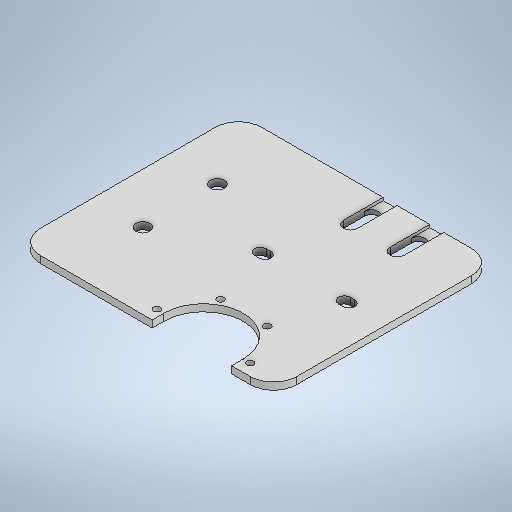
# Autodesk Inventor part: TopMount
Saved by Autodesk Inventor 2025.2 (Build 292293000, 293)
## iProperties
Created: 2025-07-18
Part Number: TopMount
Material: Generic
Document SubType Name: Modeling
Designer: Simon
Density: 1 g/cm^3
Appearance: Default
Author: Simon
Autodesk Inventor part; units mm, degrees
ref_plane "YZ Plane" through (0, 0, 0) normal (1, 0, 0) x (0, 1, 0)
ref_plane "XZ Plane" through (0, 0, 0) normal (0, 1, 0) x (-1, 0, 0)
ref_plane "XY Plane" through (0, 0, 0) normal (0, 0, 1) x (1, 0, 0)
sketch "Sketch1" plane through (0, 0, 0) normal (0, 1, 0) x (-1, 0, 0)
  line L0 (-75, 47.5) -> (75, 47.5)
  line L1 (75, 47.5) -> (75, -47.5)
  line L2 (75, -47.5) -> (-75, -47.5)
  line L3 (-75, -47.5) -> (-75, 47.5)
  line L4 (-75, 47.5) -> (75, -47.5) construction
  line L5 (75, 47.5) -> (-75, -47.5) construction
  point P0 (0, 0)
  dimension "d0" = 150
  dimension "d1" = 95
  constraints: 12 end point, 2 midpoint, 2 parallel, 1 horizontal, 1 perpendicular
  measures "d0" distance of L1.end L2.end
  measures "d1" distance of L0.end L1.end
extrude "Extrusion1" add sketch "Sketch1" along normal blind 3
sketch "Sketch4" plane through (0, 3, 0) normal (0, 1, 0) x (1, 0, 0)
  line L0 (75, 47.5) -> (-75, 47.5) projected
  line L1 (-10, 47.5) -> (10, 47.5)
  line L2 (10, 47.5) -> (10, 27.5)
  line L3 (-10, 47.5) -> (-10, 27.5)
  line L4 (-10, 27.5) -> (10, 27.5)
  line L5 (-13, 47.5) -> (-7, 47.5)
  line L6 (7, 47.5) -> (13, 47.5)
  line L7 (-10, 47.5) -> (-10, 42.5)
  line L8 (10, 47.5) -> (10, 42.5)
  line L9 (-10, 42.5) -> (-10, 39.5)
  line L10 (10, 42.5) -> (10, 39.5)
  line L11 (-10, 27.5) -> (-10, 30.5)
  line L12 (10, 27.5) -> (10, 30.5)
  circle A0 centre (-10, 30.5) radius 3
  circle A1 centre (10, 30.5) radius 3
  circle A2 centre (-10, 39.5) radius 3
  circle A3 centre (10, 39.5) radius 3
  line L13 (-13, 39.5) -> (-13, 30.5)
  line L14 (-7, 39.5) -> (-7, 30.5)
  line L15 (7, 39.5) -> (7, 30.5)
  line L16 (13, 39.5) -> (13, 30.5)
  line L17 (-10, 27.5) -> (-7, 27.5)
  line L18 (-7, 27.5) -> (-7, 47.5)
  line L19 (-7, 47.5) -> (-10, 47.5)
  line L20 (-10, 47.5) -> (-10, 27.5)
  line L21 (-10, 47.5) -> (-13, 47.5)
  line L22 (-13, 47.5) -> (-13, 27.5)
  line L23 (-13, 27.5) -> (-10, 27.5)
  line L24 (-10, 27.5) -> (-10, 47.5)
  line L25 (10, 27.5) -> (7, 27.5)
  line L26 (7, 27.5) -> (7, 47.5)
  line L27 (7, 47.5) -> (10, 47.5)
  line L28 (10, 47.5) -> (10, 27.5)
  line L29 (10, 27.5) -> (13, 27.5)
  line L30 (13, 27.5) -> (13, 47.5)
  line L31 (13, 47.5) -> (10, 47.5)
  line L32 (10, 47.5) -> (10, 27.5)
  point P0 (0, 0)
  point P1 (0, 47.5)
  point P2 (7, 47.5)
  point P3 (7, 39.5)
  point P4 (-7, 39.5)
  point P5 (-7, 47.5)
  point P6 (-13, 47.5)
  point P7 (-13, 39.5)
  dimension "d14" = 20
  dimension "d15" = 20
  dimension "d16" = 6
  dimension "d17" = 6
  dimension "d18" = 5
  dimension "d19" = 5
  dimension "d20" = 3
  dimension "d21" = 3
  dimension "d22" = 3
  dimension "d23" = 3
  constraints: 64 end point, 12 point on circle, 10 point on line, 8 parallel, 8 tangent, 6 perpendicular, 4 centre point, 4 coincident, 4 horizontal, 4 midpoint, 1 vertical
  measures "d14" distance of L1.start L1.end
  measures "d15" distance of L1.end L2.end
  measures "d16" distance of L5.start L5.end
  measures "d17" distance of L6.start L6.end
  measures "d18" distance of L1.start L7.end
  measures "d19" distance of L1.end L8.end
  measures "d20" distance of L7.end L9.end
  measures "d21" distance of L8.end L10.end
  measures "d22" distance of L3.end L11.end
  measures "d23" distance of L2.end L12.end
extrude "Extrusion3" cut sketch "Sketch4" against normal through all contours A3 L2 | L16 A1 L2 A3 | L2 A3 | L2 A1 L15 A3 | A1 L2 | L2 A1 | A2 L3 | L14 A0 L3 A2 | L3 A2 | L3 A0 L13 A2 | A0 L3 | L3 A0
extrude "Extrusion5" cut sketch "Sketch4" against normal blind 1.2 contours L30 A3 L2 L0 | L2 A3 L26 L0 | L18 A2 L3 L0 | L3 A2 L22 L0
sketch "Sketch6" plane through (0, 3, 0) normal (0, 1, 0) x (1, 0, 0)
  line L0 (75, 47.5) -> (-75, 47.5) projected
  line L1 (0, 47.5) -> (0, 22.5)
  line L2 (0, 22.5) -> (0, -20.7)
  line L3 (0, -20.7) -> (0, 0.9)
  line L4 (0, 0.9) -> (-53.4, 0.9)
  line L5 (-53.4, -15.1) -> (-53.4, 16.9)
  circle A0 centre (-53.4, 16.9) radius 3
  circle A1 centre (-53.4, -15.1) radius 3
  line L6 (-19, 0.9) -> (19, 0.9)
  circle A2 centre (19, 0.9) radius 2.5
  circle A3 centre (-19, 0.9) radius 2.5
  line L7 (-19, 0.9) -> (-17, 0.9)
  line L8 (19, 0.9) -> (17, 0.9)
  circle A4 centre (17, 0.9) radius 2.5
  circle A5 centre (-17, 0.9) radius 2.5
  line L9 (-19, 3.4) -> (-17, 3.4)
  line L10 (-19, -1.6) -> (-17, -1.6)
  line L11 (17, 3.4) -> (19, 3.4)
  line L12 (17, -1.6) -> (19, -1.6)
  point P0 (0, 0)
  dimension "d40" = 25
  dimension "d41" = 43.2
  dimension "d42" = 53.4
  dimension "d43" = 32
  dimension "d44" = 6
  dimension "d45" = 6
  dimension "d46" = 38
  dimension "d47" = 5
  dimension "d48" = 5
  dimension "d49" = 2
  dimension "d50" = 2
  dimension "d51" = 5
  dimension "d52" = 5
  constraints: 24 end point, 8 point on circle, 8 tangent, 6 centre point, 6 coincident, 4 midpoint, 3 point on line, 2 vertical, 1 horizontal, 1 perpendicular
  measures "d40" distance of L1.start L1.end
  measures "d41" distance of L1.end L2.end
  measures "d42" distance of L3.end L4.end
  measures "d43" distance of L5.start L5.end
  measures "d44" diameter of A0
  measures "d45" diameter of A1
  measures "d46" distance of L6.start L6.end
  measures "d47" diameter of A2
  measures "d48" diameter of A3
  measures "d49" distance of L7.start L7.end
  measures "d50" distance of L8.start L8.end
  measures "d51" diameter of A4
  measures "d52" diameter of A5
extrude "Extrusion6" cut sketch "Sketch6" against normal through all
sketch "Sketch7" plane through (0, 3, 0) normal (0, 1, 0) x (1, 0, 0)
  line L0 (75, 47.5) -> (-75, 47.5) projected
  line L1 (-75, -47.5) -> (75, -47.5) projected
  line L2 (75, 47.5) -> (35, 47.5)
  line L3 (35, 47.5) -> (35, -47.5)
  line L4 (35, -47.5) -> (75, -47.5)
  line L5 (75, -47.5) -> (75, 47.5)
  point P0 (0, 0)
  point P1 (75, -47.5)
  dimension "d55" = 40
  constraints: 8 end point, 2 parallel, 1 horizontal, 1 perpendicular, 1 point on line
  measures "d55" distance of L4.end L3.end
extrude "Extrusion7" cut sketch "Sketch7" against normal through all
sketch "Sketch8" plane through (0, 3, 0) normal (0, 1, 0) x (1, 0, 0)
  line L0 (-75, -47.5) -> (35, -47.5) projected
  line L1 (7, 47.5) -> (-7, 47.5) projected
  line L2 (0, 47.5) -> (0, -42.5)
  circle A0 centre (0, -42.5) radius 25
  circle A1 centre (0, -42.5) radius 20
  line L3 (0, -42.5) -> (-20, -42.5)
  circle A2 centre (-20, -42.5) radius 1.5
  circle A3 centre (-10, -59.8205) radius 1.5
  circle A4 centre (10, -59.8205) radius 1.5
  circle A5 centre (20, -42.5) radius 1.5
  circle A6 centre (10, -25.1795) radius 1.5
  circle A7 centre (-10, -25.1795) radius 1.5
  circle A8 centre (0, -42.5) radius 17
  line L4 (-17, -42.5) -> (-17, -47.5)
  line L5 (17, -42.5) -> (17, -47.5)
  point P0 (0, 0)
  dimension "d60" = 90
  dimension "d61" = 50
  dimension "d62" = 40
  dimension "d63" = 20
  dimension "d64" = 3
  dimension "d67" = 360
  dimension "d69" = 34
  constraints: 9 centre point, 9 coincident, 8 end point, 3 perpendicular, 2 point on circle, 2 point on line, 2 tangent, 1 horizontal, 1 midpoint, 19 other
  measures "d60" distance of L2.start L2.end
  measures "d61" diameter of A0
  measures "d62" diameter of A1
  measures "d63" distance of L3.start L3.end
  measures "d64" diameter of A2
  measures "d69" diameter of A8
extrude "Extrusion8" cut sketch "Sketch8" against normal through all contours L4 A8 L0 | A2 A1 | A1 L3 A2 | A8 L3 L2 L0 | A8 L2 L3 | A1 A2 L3 | A6 A1 | A1 A6 | A7 A1 | A1 A7 | L0 A8 L5 | A5 A1 | A1 A5
fillet "Fillet1" radius 10 4 edges at (35, 1.5, 47.5) (35, 1.5, -47.5) (-75, 1.5, 47.5) (-75, 1.5, -47.5)
body "Solid1"
